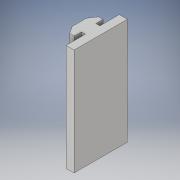
# Autodesk Inventor part: slotMountingPlate
Saved by Autodesk Inventor 2018 (Build 220112000, 112)
## iProperties
Created: 2020-03-14
Part Number: slotMountingPlate
Material: Generic
Document SubType Name: Modeling
Designer: natha
Density: 1 g/cm^3
Appearance: Default
Author: natha
Autodesk Inventor part; units mm, degrees
ref_plane "YZ Plane" through (0, 0, 0) normal (1, 0, 0) x (0, 1, 0)
ref_plane "XZ Plane" through (0, 0, 0) normal (0, 1, 0) x (-1, 0, 0)
ref_plane "XY Plane" through (0, 0, 0) normal (0, 0, 1) x (1, 0, 0)
sketch "Sketch1" plane through (0, 0, 0) normal (0, 1, 0) x (-1, 0, 0)
  line L0 (0, -5.4) -> (1.5, -5.4)
  line L1 (1.5, -5.4) -> (1.5, -8.1)
  line L2 (1.5, -8.1) -> (3.2, -8.1)
  line L3 (0, 0) -> (1.5, 0)
  line L4 (1.5, 0) -> (1.5, 2.7)
  line L5 (1.5, 2.7) -> (3.2, 2.7)
  line L6 (5, 0) -> (5, -5.4)
  line L7 (5, -5.4) -> (3.2, -8.1)
  line L8 (5, 0) -> (3.2, 2.7)
  line L9 (0, -5.4) -> (0, -12.7)
  line L10 (0, -12.7) -> (-3, -12.7)
  line L11 (-3, -12.7) -> (-3, 7.3)
  line L12 (-3, 7.3) -> (0, 7.3)
  line L13 (0, 7.3) -> (0, 0)
  dimension "d0" = 5.4
  dimension "d1" = 1.5
  dimension "d2" = 2.7
  dimension "d3" = 1.7
  dimension "d4" = 2.7
  dimension "d5" = 1.7
  dimension "d9" = 3
  dimension "d10" = 20
  dimension "d11" = 7.3
  constraints: 28 end point, 8 perpendicular, 2 vertical, 1 horizontal, 1 point on line
  measures "d0" distance of L3.start L0.start
  measures "d1" distance of L0.start L0.end
  measures "d2" distance of L0.end L1.end
  measures "d3" distance of L1.end L2.end
  measures "d4" distance of L3.end L4.end
  measures "d5" distance of L4.end L5.end
  measures "d9" distance of L9.end L10.end
  measures "d10" distance between parallel lines of L10 L12
  measures "d11" distance between parallel lines of L3 L12
extrude "Extrusion1" add sketch "Sketch1" along normal blind 40
body "Solid1"
